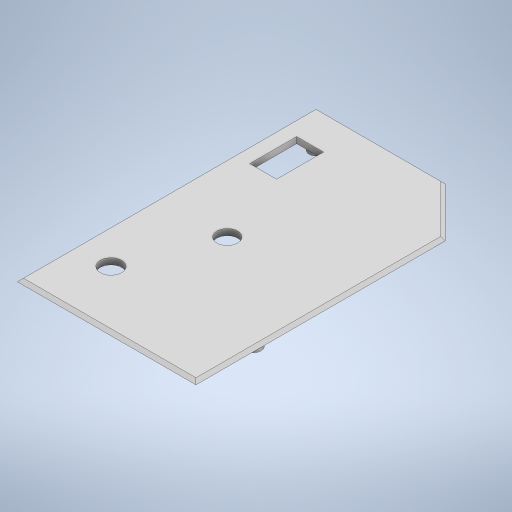
# Autodesk Inventor part: control plate
Saved by Autodesk Inventor 2024 (Build 280153000, 153)
## iProperties
Created: 2024-01-23
Part Number: control plate
Material: Generic
Document SubType Name: Modeling
Designer: Brian
Density: 1 g/cm^3
Appearance: Default
Author: Brian
Autodesk Inventor part; units mm, degrees
ref_plane "YZ Plane" through (0, 0, 0) normal (1, 0, 0) x (0, 1, 0)
ref_plane "XZ Plane" through (0, 0, 0) normal (0, 1, 0) x (-1, 0, 0)
ref_plane "XY Plane" through (0, 0, 0) normal (0, 0, 1) x (1, 0, 0)
sketch "Sketch1" plane through (0, 0, 0) normal (0, 1, 0) x (-1, 0, 0)
  line L0 (0, 0) -> (52, 0)
  line L1 (52, 0) -> (52, 91)
  line L2 (52, 91) -> (0, 91)
  line L3 (0, 91) -> (0, 0)
  circle A0 centre (43.1, 75.5) radius 3.5
  circle A1 centre (32.5, 48.34) radius 3.4
  line L4 (49.5, 24.05) -> (40.75, 24.05)
  line L5 (40.75, 24.05) -> (40.75, 8.8)
  line L6 (40.75, 8.8) -> (49.5, 8.8)
  line L7 (49.5, 8.8) -> (49.5, 24.05)
  circle A2 centre (4.5, 67.85) radius 1.75
  circle A3 centre (49.5, 2.5) radius 1.75
  point P0 (26, 0)
  dimension "d0" = 52
  dimension "d1" = 91
  dimension "d2" = 7
  dimension "d3" = 6.8
  dimension "d4" = 3.5
  dimension "d5" = 75.5
  dimension "d6" = 8.9
  dimension "d7" = 19.5
  dimension "d8" = 48.34
  dimension "d9" = 15.25
  dimension "d10" = 8.75
  dimension "d11" = 8.8
  dimension "d12" = 2.5
  dimension "d13" = 2.5
  dimension "d14" = 2.5
  dimension "d15" = 47.5
  dimension "d16" = 67.85
  constraints: 16 end point, 4 centre point, 4 parallel, 2 horizontal, 2 perpendicular, 1 equal radius, 1 midpoint
  measures "d0" distance of L1.end L2.end
  measures "d1" distance of L0.end L1.end
  measures "d2" diameter of A0
  measures "d3" diameter of A1
  measures "d4" diameter of A2
  measures "d5" distance from line of L0 A0.centre
  measures "d6" distance from line of L1 A0.centre
  measures "d7" distance from line of L1 A1.centre
  measures "d8" vertical distance of point (26, 0) A1.centre
  measures "d9" distance of L4.end L5.end
  measures "d10" distance of L4.start L4.end
  measures "d11" distance between parallel lines of L0 L6
  measures "d12" distance between parallel lines of L1 L7
  measures "d13" distance from line of L0 A3.centre
  measures "d14" distance from line of L1 A3.centre
  measures "d15" distance from line of L1 A2.centre
  measures "d16" distance from line of L0 A2.centre
extrude "Extrusion1" add sketch "Sketch1" along normal blind 2
sketch "Sketch2" plane through (0, 0, 0) normal (0, 1, 0) x (1, 0, 0)
  circle A0 centre (-4.5, -67.85) radius 2.54
  circle A1 centre (-49.5, -2.5) radius 2.286
  line L0 (-40.75, -24.05) -> (-49.5, -24.05) projected
  line L1 (-49.5, -24.05) -> (-49.5, -8.8) projected
  line L2 (-49.5, -8.8) -> (-40.75, -8.8) projected
  line L3 (-40.75, -8.8) -> (-40.75, -24.05) projected
  circle A2 centre (-49.5, -2.5) radius 1.75 projected
  circle A3 centre (-4.5, -67.85) radius 1.75 projected
  circle A4 centre (-32.5, -48.34) radius 3.4 projected
  circle A5 centre (-43.1, -75.5) radius 3.5 projected
  line L4 (0, 0) -> (-52, 0) projected
  line L5 (-52, 0) -> (-52, -91) projected
  line L6 (-52, -91) -> (0, -91) projected
  line L7 (0, -91) -> (0, 0) projected
  dimension "d19" = 5.08
  dimension "d20" = 4.572
  constraints: 2 centre point, 2 coincident
  measures "d19" diameter of A0
  measures "d20" diameter of A1
extrude "Extrusion2" add sketch "Sketch2" against normal blind 5 contours A0 | A1
sketch "Sketch3" plane through (0, 2, 0) normal (0, -1, 0) x (1, 0, 0)
  line L0 (-49.5, 24.05) -> (-40.75, 24.05) projected
  line L1 (-40.75, 24.05) -> (-40.75, 8.8) projected
  line L2 (-40.75, 8.8) -> (-49.5, 8.8) projected
  line L3 (-49.5, 8.8) -> (-49.5, 24.05) projected
  circle A0 centre (-49.5, 2.5) radius 1.75 projected
  circle A1 centre (-4.5, 67.85) radius 1.75 projected
  circle A2 centre (-32.5, 48.34) radius 3.4 projected
  circle A3 centre (-43.1, 75.5) radius 3.5 projected
  line L4 (-52, 0) -> (0, 0) projected
  line L5 (0, 0) -> (0, 91) projected
  line L6 (0, 91) -> (-52, 91) projected
  line L7 (-52, 91) -> (-52, 0) projected
extrude "Extrusion3" add sketch "Sketch3" along normal blind 0.5 contours A0 | A1
fillet "Fillet1" radius 3.175 2 edges at (-51.786, 0, 2.5) (-7.04, 0, 67.85)
sketch "Sketch4" plane through (0, 2, 0) normal (0, 1, 0) x (1, 0, 0)
  line L0 (-52, -91) -> (0, -91) projected
  line L1 (0, -91) -> (-52, -91)
  line L2 (-52, -91) -> (-52, 0)
  line L3 (-52, 0) -> (0, 0)
  line L4 (0, 0) -> (0, -91)
  line L5 (3, -94) -> (-55, -94)
  line L6 (-55, -94) -> (-55, 3)
  line L7 (-55, 3) -> (3, 3)
  line L8 (3, 3) -> (3, -94)
  point P0 (0, 0)
  dimension "d26" = 3
  constraints: 16 end point, 4 parallel, 2 perpendicular, 1 horizontal, 3 other
  measures "d26" distance between parallel lines of L4 L8
extrude "Extrusion4" add sketch "Sketch4" against normal blind 1
sketch "Sketch6" plane through (0, 2, 0) normal (0, 1, 0) x (1, 0, 0)
  line L0 (-16.05, 3) -> (3, -16.05)
  line L1 (3, -94) -> (3, 3) projected
  line L2 (-55, 3) -> (3, 3) projected
  line L3 (-16.05, 3) -> (3, 3)
  line L4 (3, 3) -> (3, -16.05)
  point P0 (0, 0)
  dimension "d32" = 19.05
  dimension "d33" = 19.05
  constraints: 6 end point, 2 collinear, 1 point on line
  measures "d32" distance of L1.end L0.end
  measures "d33" distance from line of L1 L0.start
extrude "Extrusion5" cut sketch "Sketch6" against normal blind 2
sketch "Sketch8" plane through (0, 2, 0) normal (0, 1, 0) x (1, 0, 0)
  line L0 (-16.05, 3) -> (-13.05, 0) projected
  line L1 (-16.05, 3) -> (-13.05, 3)
  line L2 (-13.05, 3) -> (2.9846, -13.0346)
  line L3 (2.9846, -13.0346) -> (2.9846, -16.0346)
  line L4 (2.9846, -16.0346) -> (-16.05, 3)
  line L5 (-16.05, 3) -> (3, -16.05) projected
  line L6 (3, -16.05) -> (3, -94) projected
  line L7 (3, -94) -> (-55, -94) projected
  line L8 (-55, -94) -> (-55, 3) projected
  line L9 (-55, 3) -> (-16.05, 3) projected
  line L10 (-49.5, -24.05) -> (-40.75, -24.05) projected
  line L11 (-40.75, -24.05) -> (-40.75, -8.8) projected
  line L12 (-40.75, -8.8) -> (-49.5, -8.8) projected
  line L13 (-49.5, -8.8) -> (-49.5, -24.05) projected
  circle A0 centre (-32.5, -48.34) radius 3.4 projected
  circle A1 centre (-43.1, -75.5) radius 3.5 projected
  point P0 (0, 0)
  point P1 (-13.05, 0)
  dimension "d36" = 3
  dimension "d37" = 3
  constraints: 8 end point, 1 collinear, 1 horizontal, 1 perpendicular
  measures "d36" distance of L2.end L3.end
  measures "d37" distance of L0.start L1.end
extrude "Extrusion6" add sketch "Sketch8" against normal blind 1 contours L1 L2 L3 L4 L0
chamfer "Chamfer1" distance 1 angle 45 5 edges at (-34.025, 2, -3) (3, 2, 55.025) (-55, 2, 45.5) (-26, 2, 94) (-5.0327, 2, 5.0173)
equation "\"d14\" = d13"
equation "\"d32\" = d33"
body "Solid1"
